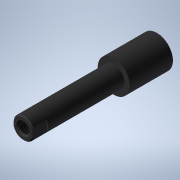
# Autodesk Inventor part: 5267300 AEN-S-6-5-I-A---(highP)
Saved by Autodesk Inventor 2021 (Build 250183000, 183)
## iProperties
Created: 2025-06-16
Part Number: 5267300 AEN-S-6-5-I-A---(highP)
Material: Generic
Catalog Web Link: www.cadenas.de
Description: AEN-S---(P)-Compact cylinder
Vendor: FESTO
Document SubType Name: Modeling
Designer: psAdmin
Manufacturer: FESTO
Mass: 0.420795 g
Surface Area: 4.58854 cm^2
Volume: 0.420795 cm^3
Density: 1 g/cm^3
Appearance: PSOLRGB-175-175-175
Category: PARTsolutions
Company: FESTO
Title: 5267300 AEN-S-6-5-I-A---(highP)
Author: Cadenas PARTsolutions
Comments: Compact cylinder
PSOL_IDENT_0: {$CADENAS_DATA/23d-libs/festo/parts/a/aen/parts/aen_s_piston.prj},215 {VTYP=3D},{NB=5267300 AEN-S-6-
PSOL_IDENT_1: 5-I-A---(highP)},{LINA=5267300 AEN-S-6-5-I-A---(highP)},{NN=AEN-S---(P)},{DATE=04.06.2025 19:32:15},
PSOL_IDENT_2: {GEOMDATE=23.08.2023 14:28:27},{VERSION=},{LINEID=30},{WBVAR=LODLEVEL},{WBNUMERIC=}  {NB=5267300 AEN
PSOL_IDENT_3: -S-6-5-I-A---(highP)},{LINA=5267300 AEN-S-6-5-I-A---(highP)},{KT=DUMMY},{TNR=5267300},{TYP=AEN-S-6-5
PSOL_IDENT_4: -I-A},{LODDEST=mechanical},{LODLEVEL=high},{LODLEVELX='high', 'High', 'medium', 'Medium','low','Low'
PSOL_IDENT_5: },{L1=17.000},{L2=25.100},{D1=6.000},{D2=4.000},{AF=5.000},{A=0.000},{SF=3.500},{KF=2.500},{KK=0.000
PSOL_IDENT_6: }
NB: 5267300 AEN-S-6-5-I-A---(highP)
NN: AEN-S---(P)
NT: Compact cylinder
NBSYN: $TNR. $TYP.---($LODLEVEL.P)
LINA: 5267300 AEN-S-6-5-I-A---(highP)
CATALOG: Festo
TNR: 5267300
TYP: AEN-S-6-5-I-A
LODLEVEL: High
L1: 17
L2: 25.1
D1: 6
D2: 4
AF: 5
A: 0
SF: 3.5
KF: 2.5
KK: 0
SUPPLIER: FESTO
ARTICLENO: 5267300 AEN-S-6-5-I-A---(highP)
BOMINFO: 5267300 AEN-S-6-5-I-A---(highP)
CREATOR: CADENAS GmbH
Autodesk Inventor part; units mm, degrees
ref_plane "YZ Plane" through (0, 0, 0) normal (1, 0, 0) x (0, 1, 0)
ref_plane "XZ Plane" through (0, 0, 0) normal (0, 1, 0) x (-1, 0, 0)
ref_plane "XY Plane" through (0, 0, 0) normal (0, 0, 1) x (1, 0, 0)
sketch "Sketch_1" plane through (0, 0, 0) normal (1, 0, 0) x (0, 1, 0)
  line L0 (0, -25.1) -> (0, -6.5811)
  line L1 (0, -6.5811) -> (1.0065, -6)
  line L2 (1.0065, -6) -> (1.0065, -0.2435)
  line L3 (1.0065, -0.2435) -> (1.25, 0)
  line L4 (1.25, 0) -> (1.8, 0)
  line L5 (1.8, 0) -> (2, -0.2)
  line L6 (2, -0.2) -> (2, -17)
  line L7 (2, -17) -> (3, -17)
  line L8 (3, -17) -> (3, -25.1)
  line L9 (3, -25.1) -> (0, -25.1)
  line L10 (0, -25.1) -> (0, -6.5811)
  constraints: 22 end point
revolve "Revolution1" add sketch "Sketch_1" angle 360 about axis through (0, 0, -25.1) along (0, 0, -1)
thread "Thread1" size "M2.5x0.45" class "6H" standard "ISO Metric profile" length 4.7565
sketch "Sketch_2" plane through (0, 0, 0) normal (0, 0, 1) x (1, 0, 0)
  line L0 (-3.5, 15) -> (-3.5, -15)
  line L1 (-3.5, -15) -> (3.5, -15)
  line L2 (3.5, -15) -> (3.5, 15)
  line L3 (3.5, 15) -> (-3.5, 15)
  line L4 (-1.75, 10) -> (-1.75, -10)
  line L5 (-1.75, -10) -> (1.75, -10)
  line L6 (1.75, -10) -> (1.75, 10)
  line L7 (1.75, 10) -> (-1.75, 10)
  constraints: 16 end point
extrude "Extrusion1" cut sketch "Sketch_2" against normal blind 2.7
ref_plane "ANBAU_XY" through (0, 0, -25.1) normal (0, 0, -1) x (1, 0, 0)
ref_plane "ANBAU_YZ" through (0, 0, -25.1) normal (1, 0, 0) x (0, -1, 0)
ref_plane "ANBAU_ZX" through (0, 0, -25.1) normal (0, -1, 0) x (0, 0, -1)
body "Solid1"
